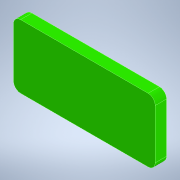
# Autodesk Inventor part: MiniUSB_ADAPTER_PCB
Saved by Autodesk Inventor 2021 (Build 250183000, 183)
## iProperties
Created: 2020-07-10
Part Number: MiniUSB_ADAPTER_PCB
Material: Generic
Document SubType Name: Modeling
Designer: lgnds
Density: 1 g/cm^3
Appearance: Default
Author: lgnds
Autodesk Inventor part; units mm, degrees
ref_plane "YZ Plane" through (0, 0, 0) normal (1, 0, 0) x (0, 1, 0)
ref_plane "XZ Plane" through (0, 0, 0) normal (0, 1, 0) x (-1, 0, 0)
ref_plane "XY Plane" through (0, 0, 0) normal (0, 0, 1) x (1, 0, 0)
sketch "Sketch1" plane through (0, 0, 0) normal (0, 0, 1) x (1, 0, 0)
  line L0 (-10, -4.5) -> (10, -4.5)
  line L1 (10, -4.5) -> (10, 4.5)
  line L2 (10, 4.5) -> (-10, 4.5)
  line L3 (-10, 4.5) -> (-10, -4.5)
  line L4 (-10, -4.5) -> (10, 4.5) construction
  line L5 (10, -4.5) -> (-10, 4.5) construction
  point P0 (0, 0)
  dimension "d0" = 20
  dimension "d1" = 9
  constraints: 12 end point, 2 midpoint, 2 parallel, 1 horizontal, 1 perpendicular
  measures "d0" distance of L1.end L2.end
  measures "d1" distance between parallel lines of L2 L0
extrude "Extrusion1" add sketch "Sketch1" along normal blind 1.6
fillet "Fillet1" radius 1 4 edges at (10, 4.5, 0.8) (-10, 4.5, 0.8) (-10, -4.5, 0.8) (10, -4.5, 0.8)
sketch "MiniUSB_ADAPTER_PCB_OUTLINE" plane through (0, 0, 1.6) normal (0, 0, 1) x (1, 0, 0)
  line L0 (3.8, 0.85) -> (3.8, 2.35) projected
  line L1 (3.5, 2.35) -> (3.5, 0.85) projected
  line L2 (3.5, 0.85) -> (3.8, 0.85) projected
  line L3 (3.8, 2.35) -> (3.5, 2.35) projected
  line L4 (-3.5, 2.35) -> (-3.5, 0.85) projected
  line L5 (-3.8, 0.85) -> (-3.8, 2.35) projected
  line L6 (-3.5, 0.85) -> (-3.8, 0.85) projected
  line L7 (-3.8, 2.35) -> (-3.5, 2.35) projected
  line L8 (-1.8, 0.175) -> (-1.4, 0.175) projected
  line L9 (-1.4, 0.175) -> (-1.4, 0.425) projected
  line L10 (-1.4, 0.425) -> (-1.8, 0.425) projected
  line L11 (-1.8, 0.425) -> (-1.8, 0.175) projected
  line L12 (0.6, 2.775) -> (1, 2.775) projected
  line L13 (1, 3.025) -> (0.6, 3.025) projected
  line L14 (0.6, 3.025) -> (0.6, 2.775) projected
  line L15 (1, 2.775) -> (1, 3.025) projected
  line L16 (1.875, -1.1641) -> (-1.875, -1.1641) projected
  line L17 (1.4, 0.175) -> (1.8, 0.175) projected
  line L18 (1.8, 0.425) -> (1.4, 0.425) projected
  line L19 (1.4, 0.425) -> (1.4, 0.175) projected
  line L20 (1.8, 0.175) -> (1.8, 0.425) projected
  line L21 (-1, 2.775) -> (-0.6, 2.775) projected
  line L22 (-1, 3.025) -> (-1, 2.775) projected
  line L23 (-0.6, 3.025) -> (-1, 3.025) projected
  line L24 (-0.6, 2.775) -> (-0.6, 3.025) projected
  line L25 (0.2, 0.425) -> (-0.2, 0.425) projected
  line L26 (0.2, 0.175) -> (0.2, 0.425) projected
  line L27 (-0.2, 0.175) -> (0.2, 0.175) projected
  line L28 (-0.2, 0.425) -> (-0.2, 0.175) projected
  circle A0 centre (-3.65, 1.6) radius 0.75
  circle A1 centre (3.65, 1.6) radius 0.75
  arc A2 (9, -4.5) -> (10, -3.5) centre (9, -3.5) ccw projected
  line L29 (10, -3.5) -> (10, 3.5) projected
  arc A3 (10, 3.5) -> (9, 4.5) centre (9, 3.5) ccw projected
  line L30 (9, 4.5) -> (-9, 4.5) projected
  arc A4 (-9, 4.5) -> (-10, 3.5) centre (-9, 3.5) ccw projected
  line L31 (-10, 3.5) -> (-10, -3.5) projected
  arc A5 (-10, -3.5) -> (-9, -4.5) centre (-9, -3.5) ccw projected
  line L32 (-9, -4.5) -> (9, -4.5) projected
  point P0 (0, 0)
  constraints: 2 centre point
body "Solid1"
